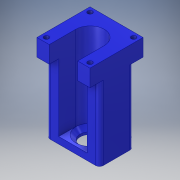
# Autodesk Inventor part: Lower_Unit
Saved by Autodesk Inventor 2019 (Build 230136000, 136)
## iProperties
Created: 2018-10-09
Part Number: Lower_Unit
Material: Generisch
Document SubType Name: Modeling
Designer: janbe
Density: 1 g/cm^3
Appearance: Blau - Wandfarbe - glänzend
Author: janbe
Autodesk Inventor part; units mm, degrees
ref_plane "YZ Plane" through (0, 0, 0) normal (1, 0, 0) x (0, 1, 0)
ref_plane "XZ Plane" through (0, 0, 0) normal (0, 1, 0) x (-1, 0, 0)
ref_plane "XY Plane" through (0, 0, 0) normal (0, 0, 1) x (1, 0, 0)
sketch "Skizze1" plane through (0, 0, 0) normal (0, 1, 0) x (-1, 0, 0)
  arc A0 (-7.5, 0) -> (7.5, 0) centre (0, 0) ccw
  line L0 (-14, 14) -> (-14, -14)
  line L1 (-14, -14) -> (14, -14)
  line L2 (14, -14) -> (14, 14)
  line L3 (7.5, 0) -> (7.5, 14)
  line L4 (-7.5, 0) -> (-7.5, 14)
  line L5 (14, 14) -> (7.5, 14)
  line L6 (-7.5, 14) -> (-14, 14)
  dimension "d0" = 15
  dimension "d1" = 28
  dimension "d2" = 28
  dimension "d3" = 14
  dimension "d4" = 14
  constraints: 14 end point, 4 parallel, 4 perpendicular, 2 horizontal, 2 point on circle, 2 tangent, 1 centre point, 1 coincident, 1 collinear
  measures "d0" diameter of A0
  measures "d1" distance of L1.end L2.end
  measures "d2" distance of L0.end L1.end
  measures "d3" distance from line of L2 point (0, 0)
  measures "d4" distance from line of L1 point (0, 0)
extrude "Extrusion1" add sketch "Skizze1" against normal blind 49.5
sketch "Skizze2" plane through (0, -49.5, 0) normal (0, -1, 0) x (1, 0, 0)
  line L0 (-14, 14) -> (-14, -14) projected
  line L1 (-14, -14) -> (14, -14) projected
  line L2 (14, -14) -> (14, 14) projected
  line L3 (14, 14) -> (7.5, 14) projected
  line L4 (7.5, 14) -> (7.5, 0) projected
  arc A0 (-7.5, 0) -> (7.5, 0) centre (0, 0) ccw projected
  line L5 (-7.5, 0) -> (-7.5, 14) projected
  line L6 (-7.5, 14) -> (-14, 14) projected
  line L7 (-7.5, 0) -> (-7.5, 14) projected
  line L8 (-7.5, 14) -> (7.5, 14)
  circle A1 centre (0, 0) radius 5.2
  dimension "d7" = 10.4
  constraints: 2 end point, 1 centre point, 1 coincident, 1 perpendicular
  measures "d7" diameter of A1
extrude "Extrusion2" add sketch "Skizze2" against normal blind 5 contours L8 L4 A0 L5
chamfer "Fase1" distance 2.25 angle 45 1 edges at (-5.2, -44.5, 0)
sketch "Skizze5" plane through (0, 0, 0) normal (0, 1, 0) x (1, 0, 0)
  circle A0 centre (-11.5, -11.5) radius 1.25
  line L0 (-14, -14) -> (-14, 14) projected
  line L1 (-7.5, -14) -> (-14, -14) projected
  line L2 (-7.5, 0) -> (-7.5, -14) projected
  arc A1 (7.5, 0) -> (-7.5, 0) centre (0, 0) ccw projected
  line L3 (7.5, -14) -> (7.5, 0) projected
  line L4 (14, -14) -> (7.5, -14) projected
  line L5 (14, 14) -> (14, -14) projected
  line L6 (-14, 14) -> (14, 14) projected
  circle A2 centre (11.5, -11.5) radius 1.25
  circle A3 centre (-11.5, 11.5) radius 1.25
  circle A4 centre (11.5, 11.5) radius 1.25
  dimension "d21" = 2.5
  dimension "d22" = 2.5
  dimension "d23" = 2.5
  dimension "d26" = 23
  dimension "d29" = 23
  constraints: 4 centre point, 1 horizontal, 1 vertical, 6 other
  measures "d21" diameter of A0
  measures "d22" distance from line of A0.centre L1
  measures "d23" distance from line of L0 A0.centre
  measures "d26" distance of A0.centre A2.centre
  measures "d29" distance of A0.centre A3.centre
extrude "Extrusion5" cut sketch "Skizze5" against normal blind 50 contours A0 | A2 | A3 | A4
sketch "Skizze7" plane through (0, -49.5, 0) normal (0, -1, 0) x (1, 0, 0)
  circle A0 centre (-11.5, 11.5) radius 1.25 projected
  circle A1 centre (0, 0) radius 5.2 projected
  line L0 (-14, 14) -> (-14, -14) projected
  line L1 (-14, -14) -> (14, -14) projected
  line L2 (14, -14) -> (14, 14) projected
  line L3 (14, 14) -> (-14, 14) projected
  circle A2 centre (11.5, 11.5) radius 1.25 projected
  circle A3 centre (11.5, -11.5) radius 1.25 projected
  circle A4 centre (-11.5, -11.5) radius 1.25 projected
  line L4 (14, -14) -> (14, 14) projected
  line L5 (14, 14) -> (9, 14)
  line L6 (9, 14) -> (9, 9)
  line L7 (9, 9) -> (14, 9)
  line L8 (14, 9) -> (14, 14)
  line L9 (-14, 14) -> (-9, 14)
  line L10 (-9, 14) -> (-9, 9)
  line L11 (-9, 9) -> (-14, 9)
  line L12 (-14, 9) -> (-14, 14)
  line L13 (-14, -14) -> (-9, -14)
  line L14 (-9, -14) -> (-9, -9)
  line L15 (-9, -9) -> (-14, -9)
  line L16 (-14, -9) -> (-14, -14)
  line L17 (14, -14) -> (9, -14)
  line L18 (9, -14) -> (9, -9)
  line L19 (9, -9) -> (14, -9)
  line L20 (14, -9) -> (14, -14)
  line L21 (9, 9) -> (-9, 9)
  line L22 (-9, 9) -> (-9, 14)
  line L23 (-9, 14) -> (9, 14)
  line L24 (9, 14) -> (9, 9)
  dimension "d45" = 5
  dimension "d46" = 5
  dimension "d47" = 5
  dimension "d48" = 5
  dimension "d49" = 5
  dimension "d50" = 5
  constraints: 40 end point, 10 parallel, 5 horizontal, 5 perpendicular, 2 point on line
  measures "d45" distance of L7.end L6.end
  measures "d46" distance of L6.end L5.end
  measures "d47" distance of L10.end L11.end
  measures "d48" distance of L14.end L13.end
  measures "d49" distance of L18.end L19.end
  measures "d50" distance of L17.end L18.end
extrude "Extrusion7" cut sketch "Skizze7" against normal blind 40.5 contours A0 | L3 L10 L11 L0 | L3 L6 L21 L10 | L15 L14 L1 L0 | L3 L2 L7 L6 | L18 L19 L2 L1 | A2 | A3 | A4
fillet "Rundung3" radius 2 6 edges at (14, -29.25, 9) (14, -29.25, -9) (-14, -29.25, 9) (9, -29.25, -14) (-9, -29.25, -14) (-14, -29.25, -9)
sketch "Skizze8" plane through (0, -49.5, 0) normal (0, -1, 0) x (1, 0, 0)
  circle A0 centre (0, 0) radius 5.2 projected
  arc A1 (-14, -7) -> (-12, -9) centre (-12, -7) ccw projected
  line L0 (-12, -9) -> (-9, -9) projected
  line L1 (-9, -9) -> (-9, -12) projected
  arc A2 (-9, -12) -> (-7, -14) centre (-7, -12) ccw projected
  line L2 (-7, -14) -> (7, -14) projected
  arc A3 (7, -14) -> (9, -12) centre (7, -12) ccw projected
  line L3 (9, -12) -> (9, -9) projected
  line L4 (9, -9) -> (12, -9) projected
  arc A4 (12, -9) -> (14, -7) centre (12, -7) ccw projected
  line L5 (14, -7) -> (14, 7) projected
  arc A5 (14, 7) -> (12, 9) centre (12, 7) ccw projected
  line L6 (12, 9) -> (-12, 9) projected
  arc A6 (-12, 9) -> (-14, 7) centre (-12, 7) ccw projected
  line L7 (-14, 7) -> (-14, -7) projected
extrude "Extrusion8" cut sketch "Skizze8" against normal blind 1.5
